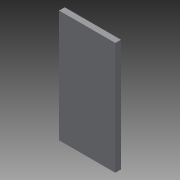
# Autodesk Inventor part: ceilplate
Saved by Autodesk Inventor 2015 (Build 190159000, 159)
## iProperties
Created: 2014-07-22
Part Number: ceilplate
Material: Generic
Document SubType Name: Modeling
Designer: shohei
Density: 1 g/cm^3
Appearance: Default
Author: shohei
Autodesk Inventor part; units mm, degrees
ref_plane "YZ Plane" through (0, 0, 0) normal (1, 0, 0) x (0, 1, 0)
ref_plane "XZ Plane" through (0, 0, 0) normal (0, 1, 0) x (-1, 0, 0)
ref_plane "XY Plane" through (0, 0, 0) normal (0, 0, 1) x (1, 0, 0)
sketch "Sketch1" plane through (0, 0, 0) normal (0, 1, 0) x (-1, 0, 0)
  line L0 (-50, 100) -> (50, 100)
  line L1 (50, 100) -> (50, -100)
  line L2 (50, -100) -> (-50, -100)
  line L3 (-50, -100) -> (-50, 100)
  line L4 (-50, 100) -> (50, -100) construction
  line L5 (50, 100) -> (-50, -100) construction
  point P0 (0, 0)
  dimension "d0" = 100
  dimension "d1" = 200
  constraints: 12 end point, 2 midpoint, 2 parallel, 1 horizontal, 1 perpendicular
  measures "d0" distance of L1.end L2.end
  measures "d1" distance of L0.end L1.end
extrude "Extrusion1" add sketch "Sketch1" along normal blind 10
body "Solid1"
